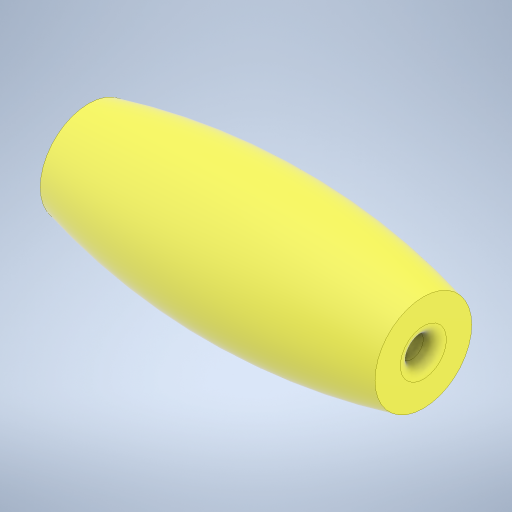
# Autodesk Inventor part: roller
Saved by Autodesk Inventor 2024.2 (Build 282272000, 272)
## iProperties
Created: 2024-04-01
Part Number: roller
Material: Polyethylene, Low Density
Document SubType Name: Modeling
Designer: Robin
Density: 0.894 g/cm^3
Appearance: Smooth - Off-White
Mass: 1.68631 g
Surface Area: 9.61717 cm^2
Volume: 1.88625 cm^3
Author: Robin
Autodesk Inventor part; units mm, degrees
ref_plane "YZ Plane" through (0, 0, 0) normal (1, 0, 0) x (0, 1, 0)
ref_plane "XZ Plane" through (0, 0, 0) normal (0, 1, 0) x (-1, 0, 0)
ref_plane "XY Plane" through (0, 0, 0) normal (0, 0, 1) x (1, 0, 0)
sketch "Sketch1" plane through (0, 0, 0) normal (0, 1, 0) x (-1, 0, 0)
  line L0 (14.5, 6) -> (-14.5, 6)
  line L1 (-14.5, 6) -> (-14.5, -6)
  line L2 (-14.5, -6) -> (14.5, -6)
  line L3 (14.5, -6) -> (14.5, 6)
  arc A0 (-14.5, -4.1905) -> (14.5, -4.1905) centre (0, 53) ccw
  line L4 (14.5, 0) -> (-14.5, 0)
  line L5 (20.3, 0) -> (-20.3, 0) projected
  point P0 (0, 0)
  point P1 (0, -6)
  dimension "d0" = 12
  dimension "d1" = 29
  dimension "d2" = 59
  constraints: 10 end point, 3 midpoint, 3 point on circle, 2 horizontal alignment, 2 parallel, 2 point on line, 1 centre point, 1 horizontal, 1 perpendicular, 1 vertical alignment
  measures "d0" distance of L2.end L0.start
  measures "d1" distance of L1.end L2.end
  measures "d2" radius of A0
revolve "Revolution1" add sketch "Sketch1" angle 360 about axis through (-10, 0, 0) along (1, 0, 0) contours L3 A0 L1 L4
sketch "Sketch2" plane through (14.5, 0, 0) normal (1, 0, 0) x (0, 0, -1)
  point P0 (0, 0)
  point P1 (0, 0)
  constraints: 1 coincident
hole "Hole1" at (14.5, 0, 0) direction (-1, 0, 0) diameter 2 end through all
fillet "Fillet1" radius 1 1 edges at (14.5, 0, 1)
fillet "Fillet2" radius 2 1 edges at (-14.5, 0, 1)
body "Solid1"
